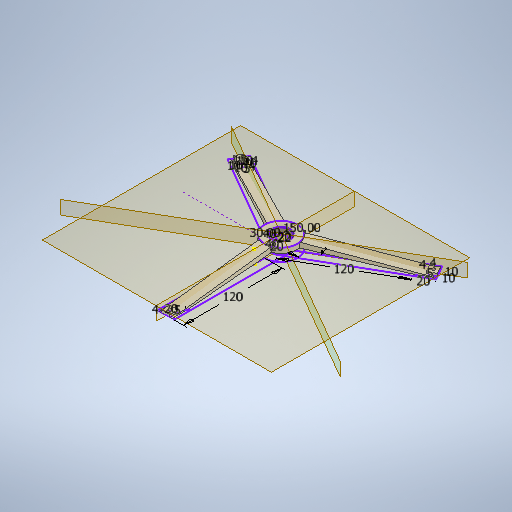
# Autodesk Inventor part: axis
Saved by Autodesk Inventor 2025 (Build 290162000, 162)
## iProperties
Created: 2025-10-01
Part Number: axis
Material: Типовые
Document SubType Name: Modeling
Designer: Admin
Density: 1 g/cm^3
Appearance: По умолчанию
Author: Admin
Autodesk Inventor part; units mm, degrees
ref_plane "YZ Plane" through (0, 0, 0) normal (1, 0, 0) x (0, 1, 0)
ref_plane "XY Plane" through (0, 0, 0) normal (0, 0, 1) x (1, 0, 0)
sketch "Эскиз1" plane through (0, 0, 0) normal (0, 1, 0) x (-1, 0, 0)
  circle A0 centre (-0.8899, -31.6552) radius 10
  circle A1 centre (-0.8899, -31.6552) radius 20
  line L0 (-0.8899, -11.6552) -> (-0.8899, 108.3448)
  line L1 (-0.8899, -31.6552) -> (78.1589, -77.294)
  line L2 (-0.8899, -31.6552) -> (90.3878, -31.6552) construction
  line L3 (78.1589, -77.294) -> (120.2106, -101.5726)
  line L4 (-0.8899, -31.6552) -> (116.9091, -31.6552) construction
  line L5 (-0.8899, -31.6552) -> (-104.8129, -91.6552)
  line L6 (-0.8899, -31.6552) -> (119.1101, -31.6552) construction
  line L7 (-104.8129, -91.6552) -> (-122.5612, -101.9021)
  line L8 (-122.5612, -101.9021) -> (-117.5612, -110.5624)
  line L9 (-117.5612, -110.5624) -> (4.1101, -40.3154)
  line L10 (-122.5612, -101.9021) -> (-127.5612, -93.2419)
  line L11 (-127.5612, -93.2419) -> (-5.8899, -22.9949)
  line L12 (120.2106, -101.5726) -> (125.2106, -92.9123)
  line L13 (125.2106, -92.9123) -> (4.1101, -22.9949)
  line L14 (120.2106, -101.5726) -> (7.7704, -36.6552)
  line L15 (-0.8899, 108.3448) -> (-10.8899, 108.3448)
  line L16 (-10.8899, 108.3448) -> (9.1101, 108.3448)
  line L17 (9.1101, 108.3448) -> (9.1101, -31.6552)
  line L18 (-10.8899, 108.3448) -> (-10.8899, -31.6552)
  line L19 (120.2106, -101.5726) -> (115.2106, -110.2328)
  line L20 (115.2106, -110.2328) -> (-5.8899, -40.3154)
  line L21 (9.1101, 108.3448) -> (9.1101, 88.3448)
  line L22 (9.1101, 88.3448) -> (-10.8899, 88.3448)
  line L23 (-10.8899, 108.3448) -> (9.1101, 88.3448)
  line L24 (9.1101, 108.3448) -> (-10.8899, 88.3448)
  line L25 (-0.8899, 98.3448) -> (-0.8899, 93.3448)
  line L26 (-0.8899, 93.3448) -> (4.1101, 93.3448)
  line L27 (4.1101, 103.3448) -> (-5.8899, 103.3448)
  line L28 (-5.8899, 103.3448) -> (-5.8899, 93.3448)
  line L29 (-5.8899, 93.3448) -> (-0.8899, 93.3448)
  line L30 (-127.5612, -93.2419) -> (-110.2407, -83.2419)
  line L31 (-110.2407, -83.2419) -> (-100.2407, -100.5624)
  line L32 (-127.5612, -93.2419) -> (-100.2407, -100.5624)
  line L33 (-117.5612, -110.5624) -> (-110.2407, -83.2419)
  line L34 (-113.9009, -96.9021) -> (-118.2311, -99.4021)
  line L35 (-118.2311, -99.4021) -> (-115.7311, -103.7322)
  line L36 (-115.7311, -103.7322) -> (-107.0708, -98.7322)
  line L37 (-107.0708, -98.7322) -> (-112.0708, -90.072)
  line L38 (-112.0708, -90.072) -> (-120.7311, -95.072)
  line L39 (-120.7311, -95.072) -> (-118.2311, -99.4021)
  circle A2 centre (-113.9009, -96.9021) radius 2
  line L40 (120.2106, -101.5726) -> (111.5503, -96.5726)
  line L41 (111.5503, -96.5726) -> (102.8901, -91.5726)
  line L42 (102.8901, -91.5726) -> (107.2202, -94.0726)
  line L43 (107.2202, -94.0726) -> (104.7202, -98.4027)
  line L44 (104.7202, -98.4027) -> (113.3805, -103.4027)
  line L45 (113.3805, -103.4027) -> (118.3805, -94.7424)
  line L46 (118.3805, -94.7424) -> (109.7202, -89.7424)
  line L47 (109.7202, -89.7424) -> (107.2202, -94.0726)
  line L48 (104.7202, -98.4027) -> (118.3805, -94.7424)
  circle A3 centre (111.5503, -96.5726) radius 2
  circle A4 centre (-118.2311, -99.4021) radius 2
  line L49 (-113.9009, -96.9021) -> (-116.2311, -92.4739)
  line L50 (-116.2311, -92.4739) -> (-125.0612, -97.572)
  line L51 (-113.9009, -96.9021) -> (-111.4009, -101.2322)
  line L52 (-111.4009, -101.2322) -> (-120.0612, -106.2322)
  line L53 (-125.0612, -97.572) -> (-120.0612, -106.2322)
  line L54 (-5.8899, 103.3448) -> (-5.8899, 108.3448)
  line L55 (4.1101, 103.3448) -> (4.1101, 108.3448)
  line L56 (4.1101, 103.3448) -> (4.1101, 98.3448)
  line L57 (4.1101, 98.3448) -> (-5.8899, 98.3448)
  circle A5 centre (-0.8899, 103.3448) radius 2
  line L58 (118.3805, -94.7424) -> (122.7106, -97.2424)
  line L59 (113.3805, -103.4027) -> (117.7106, -105.9027)
  line L60 (111.5503, -96.5726) -> (109.0503, -100.9027)
  line L61 (111.5503, -96.5726) -> (114.0503, -92.2424)
  circle A6 centre (115.8805, -99.0726) radius 2
  point P0 (0, 0)
  point P1 (-0.8899, 101.3448)
  point P2 (1.1101, 103.3448)
  point P3 (-0.8899, 103.3448)
  dimension "d0" = 20
  dimension "d1" = 40
  dimension "d2" = 120
  dimension "d3" = 30
  dimension "d4" = 120
  dimension "d5" = 150
  dimension "d6" = 10
  dimension "d7" = 10
  dimension "d8" = 10
  dimension "d9" = 10
  dimension "d13" = 20
  dimension "d38" = 5
  dimension "d39" = 20
  dimension "d40" = 5
  dimension "d41" = 4
  dimension "d42" = 10
  dimension "d43" = 10
  dimension "d44" = 5
  dimension "d45" = 10
  dimension "d46" = 10
  dimension "d47" = 10
  dimension "d48" = 4
  dimension "d53" = 4
  dimension "d58" = 4
  dimension "d63" = 4
  constraints: 124 end point, 28 point on line, 21 perpendicular, 15 midpoint, 5 centre point, 5 coincident, 4 horizontal, 2 equal length, 2 vertical, 1 collinear, 1 parallel, 1 vertical alignment, 15 other
  measures "d2" distance of L0.start L0.end
  measures "d3" angle of L1 L2
  measures "d4" distance of L1.start L5.end
  measures "d5" angle of L5 L6
  measures "d6" distance of L7.end L8.end
  measures "d7" distance of L7.end L10.end
  measures "d8" distance of L3.end L12.end
  measures "d9" distance of L14.start L19.end
  measures "d13" distance of L16.end L21.end
  measures "d38" distance of L25.start L25.end
  measures "d39" distance of L10.end L30.end
  measures "d40" distance of L34.start L34.end
  measures "d41" diameter of A2
  measures "d42" distance of L14.start L40.end
  measures "d43" distance of L40.end L41.end
  measures "d44" distance of L42.end L43.end
  measures "d45" distance of L43.end L44.end
  measures "d46" distance of L44.end L45.end
  measures "d47" distance of L45.end L46.end
  measures "d48" diameter of A3
  measures "d53" diameter of A4
  measures "d58" diameter of A5
  measures "d63" diameter of A6
ref_plane "РабПлоскость1" through (0, 15, 0) normal (0, 1, 0) x (-1, 0, 0)
sketch "Эскиз2" plane through (0, 15, 0) normal (0, 1, 0) x (-1, 0, 0)
  circle A0 centre (-0.8908, -31.6557) radius 10
  circle A1 centre (-0.8908, -31.6557) radius 20
  circle A2 centre (-0.8908, -31.6557) radius 11
  point P0 (0, 0)
  dimension "d11" = 20
  dimension "d12" = 40
  dimension "d68" = 22
  constraints: 3 centre point, 2 coincident
  measures "d11" diameter of A0
  measures "d12" diameter of A1
  measures "d68" diameter of A2
extrude "Выдавливание1" add sketch "Эскиз2" against normal blind 6 contours A1 | A2
ref_plane "РабПлоскость2" through (0.8899, 0, -31.6552) normal (0.5, 0, 0.866) x (0.866, 0, -0.5)
ref_plane "РабПлоскость3" through (-120.2106, 0, -101.5726) normal (0.5, 0, -0.866) x (0.866, 0, 0.5)
sketch "Эскиз4" plane through (0.8899, 0, -31.6552) normal (0.5, 0, 0.866) x (0.866, 0, -0.5)
  line L0 (20.0011, 15) -> (-19.9989, 15) projected
  line L1 (-19.9989, 9) -> (20.0011, 9) projected
  line L2 (20.0011, 15) -> (20.0011, 9)
  line L3 (20.0011, 15) -> (140.5253, 0)
  line L4 (140.5253, 0) -> (120.5253, 0)
  line L5 (120.5253, 0) -> (20.0011, 9)
  line L6 (20.0011, 15) -> (19.0011, 15)
  line L7 (20.0011, 15) -> (18.0011, 15)
  line L8 (18.0011, 15) -> (18.0011, 9)
  line L9 (20.0011, 9) -> (18.0011, 9)
  point P0 (-16.5982, 0)
  point P1 (-17.3194, 15)
  point P2 (-17.3194, 15)
  dimension "d22" = 20
  dimension "d25" = 2
  constraints: 16 end point, 3 point on line, 1 collinear, 1 horizontal, 1 perpendicular, 1 vertical
  measures "d22" distance of L3.end L4.end
  measures "d25" distance of L0.start L7.end
extrude "Выдавливание3" add sketch "Эскиз4" along normal mid plane 15
ref_plane "РабПлоскость4" through (0.8899, 0, -11.6552) normal (1, 0, 0) x (0, 0, 1)
sketch "Эскиз5" plane through (0.8899, 0, -11.6552) normal (1, 0, 0) x (0, 0, 1)
  point P0 (11.6552, 0)
sketch "Эскиз6" plane through (0.8899, 0, -11.6552) normal (1, 0, 0) x (0, 0, 1)
  line L0 (-40.0005, -15) -> (-0.0005, -15) projected
  line L1 (-0.0005, -15) -> (119.9781, 0)
  line L2 (119.9781, 0) -> (99.9781, 0)
  line L3 (-0.0005, -9) -> (-40.0005, -9) projected
  line L4 (99.9781, 0) -> (-0.0005, -9)
  line L5 (-0.0005, -9) -> (-2.0005, -9)
  line L6 (-2.0005, -9) -> (-2.0005, -15)
  line L7 (-0.0005, -15) -> (-2.0005, -15)
  point P0 (11.6552, 0)
  point P1 (-35.766, -15)
  point P2 (-22.7756, -15)
  point P3 (-22.7756, -9)
  point P4 (-35.766, -9)
  dimension "d29" = 20
  dimension "d30" = 2
  constraints: 12 end point, 2 point on line, 1 collinear, 1 horizontal, 1 perpendicular
  measures "d29" distance of L1.end L2.end
  measures "d30" distance of L3.start L5.end
extrude "Выдавливание4" add sketch "Эскиз6" along normal mid plane 15
sketch "Эскиз7" plane through (-120.2106, 0, -101.5726) normal (0.5, 0, -0.866) x (0.866, 0, 0.5)
  line L0 (119.8354, -15) -> (142.6104, -15) projected
  line L1 (119.8354, -15) -> (0, 0)
  line L2 (0, 0) -> (20, 0)
  line L3 (142.6104, -9) -> (119.8354, -9) projected
  line L4 (20, 0) -> (119.8354, -9)
  line L5 (119.8354, -9) -> (121.8354, -9)
  line L6 (121.8354, -9) -> (121.8354, -15)
  line L7 (119.8354, -15) -> (121.8354, -15)
  point P0 (154.8917, 0)
  point P1 (142.6094, -15)
  point P2 (142.6094, -9)
  dimension "d33" = 20
  dimension "d34" = 2
  constraints: 12 end point, 2 point on line, 1 collinear, 1 horizontal, 1 perpendicular
  measures "d33" distance of L1.end L2.end
  measures "d34" distance of L3.end L5.end
extrude "Выдавливание5" add sketch "Эскиз7" along normal mid plane 15
extrude "Выдавливание8" add sketch "Эскиз1" along normal blind 3 contours L50 L39 A4 L7 L10 | L38 L49 A2 L32 | L32 A2 L7 A4 L39 | L8 L7 A4 L35 L52 | L35 A4 L7 A2 L33 | L33 A2 L51 L36 | A2 L49 L32 | L32 L7 A2 | L33 A2 L7 | L51 A2 L33 picked at (-115.1931, -97.2034) picked at (-114.6016, -98.0289)
extrude "Выдавливание9" cut sketch "Эскиз1" along normal blind 4 contours A4 L7 L39 | L39 L7 A4 | A4 L7 L35 | L35 L7 A4
extrude "Выдавливание10" add sketch "Эскиз1" along normal blind 3 contours L55 L27 A5 L0 L16 | L56 L57 L24 | L24 L0 A5 L27 | L23 L27 A5 L0 | L57 L28 L23 | L0 A5 L27 L54 L15 | A5 L0 L27 picked at (0.232, 102.6399)
extrude "Выдавливание11" cut sketch "Эскиз1" along normal blind 3 contours A5 L0 L27 | L27 L0 A5 | A5 L27 L0 | L0 L27 A5
extrude "Выдавливание12" add sketch "Эскиз1" along normal blind 3 contours L12 L3 A6 L45 L58 | L59 L45 A6 L3 L19 | L48 A3 L61 L46 | L45 A6 L3 A3 L48 | L44 L60 A3 L3 A6 L45 | A3 L3 L48 | L48 L61 A3 | L3 A3 L60 picked at (112.8333, -96.9164)
extrude "Выдавливание13" cut sketch "Эскиз1" along normal blind 3 contours A6 L45 L3 | L3 L45 A6 | L45 L3 A6 | A6 L3 L45
sketch "Эскиз8" plane through (0, 15, 0) normal (0, 1, 0) x (1, 0, 0)
  point P0 (0, 0)
extrude "Выдавливание14" cut sketch "Эскиз2" against normal blind 10 contours A0 | A2
